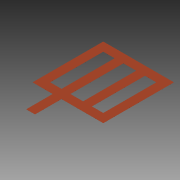
# Autodesk Inventor part: Circle_Copper
Saved by Autodesk Inventor 2014 SP1 (Build 180222100, 222)
## iProperties
Created: 2014-01-13
Part Number: Circle_Copper
Material: Copper
Document SubType Name: Modeling
Designer: tuleu
Density: 8.94 g/cm^3
Appearance: Copper - Satin
Author: tuleu
Autodesk Inventor part; units mm, degrees
ref_plane "YZ Plane" through (0, 0, 0) normal (1, 0, 0) x (0, 1, 0)
ref_plane "XZ Plane" through (0, 0, 0) normal (0, 1, 0) x (-1, 0, 0)
ref_plane "XY Plane" through (0, 0, 0) normal (0, 0, 1) x (1, 0, 0)
sketch "Sketch1" plane through (0, 0, 0) normal (0, 1, 0) x (-1, 0, 0)
  line L0 (-43.75, -43.75) -> (-43.75, 43.75)
  line L1 (-31.25, -31.25) -> (-31.25, 31.25)
  line L2 (43.75, -43.75) -> (43.75, 107.5)
  line L3 (31.25, -31.25) -> (31.25, 31.25)
  line L4 (6.25, -31.25) -> (6.25, 31.25)
  line L5 (-6.25, -31.25) -> (-6.25, 31.25)
  line L6 (31.25, -31.25) -> (6.25, -31.25)
  line L7 (-6.25, -31.25) -> (-31.25, -31.25)
  line L8 (-31.25, 31.25) -> (-6.25, 31.25)
  line L9 (6.25, 31.25) -> (31.25, 31.25)
  line L10 (31.25, 43.75) -> (31.25, 107.5)
  line L11 (31.25, 107.5) -> (43.75, 107.5)
  line L12 (-43.75, 43.75) -> (31.25, 43.75)
  line L13 (-43.75, -43.75) -> (43.75, -43.75)
  line L14 (0, -43.75) -> (0, 43.75) construction
  line L15 (-43.75, 0) -> (43.75, 0) construction
  circle A0 centre (0, 0) radius 75 construction
  point P0 (0, 0)
  dimension "d25" = 12.5
  dimension "d27" = 12.5
  dimension "d28" = 25
  dimension "d29" = 12.5
  dimension "d30" = 107.5
  constraints: 32 end point, 12 perpendicular, 6 parallel, 4 midpoint, 3 collinear, 3 horizontal, 2 point on line, 1 vertical, 3 other
  measures "d25" distance between parallel lines of L4 L5
  measures "d27" distance between parallel lines of L2 L3
  measures "d28" distance of L5.start L1.start
  measures "d29" distance between parallel lines of L12 L8
  measures "d30" distance from line of L11 A0.centre
extrude "Extrusion1" add sketch "Sketch1" along normal mid plane 0.01
body "Solid1"
